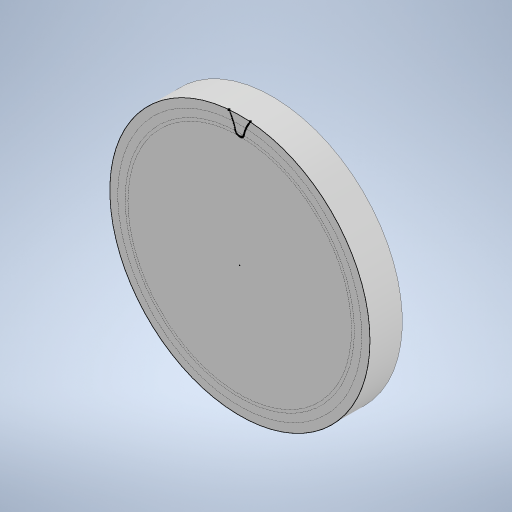
# Autodesk Inventor part: z
Saved by Autodesk Inventor 2024 (Build 280153000, 153)
## iProperties
Created: 2023-10-17
Part Number: z
Material: Generic
Document SubType Name: Modeling
Designer: Kippi
Density: 1 g/cm^3
Appearance: Default
Author: Kippi
Autodesk Inventor part; units mm, degrees
ref_plane "YZ Plane" through (0, 0, 0) normal (1, 0, 0) x (0, 1, 0)
ref_plane "XZ Plane" through (0, 0, 0) normal (0, 1, 0) x (-1, 0, 0)
ref_plane "XY Plane" through (0, 0, 0) normal (0, 0, 1) x (1, 0, 0)
sketch "Sketch1" plane through (0, 0, 0) normal (0, 0, 1) x (1, 0, 0)
  spline S0 degree 3 poles (-6.5259, 79.7334) (-6.2263, 79.2581) (-5.7769, 78.5452) (-5.2243, 77.5668) (-4.8273, 76.8235) (-4.451, 76.0694) (-4.0967, 75.3048) (-3.7666, 74.5294) (-3.4631, 73.7432) (-3.1905, 72.9457) (-2.9506, 72.1376) (-2.7945, 71.4528) (-2.6817, 70.9025) (-2.5626, 70.4977) (-2.4016, 70.1077) (-2.1917, 69.7409) (-1.9706, 69.4668) (-1.7708, 69.2687) (-1.6019, 69.1425) (-1.4288, 69.0215) (-1.2381, 68.9312) (-1.0444, 68.8474) (-0.8391, 68.7979) (-0.6323, 68.7561) (-0.3509, 68.7461) (0, 68.7526) (0.3509, 68.7461) (0.6323, 68.7561) (0.8391, 68.7979) (1.0444, 68.8474) (1.2381, 68.9312) (1.4288, 69.0215) (1.6019, 69.1425) (1.7708, 69.2687) (1.9706, 69.4668) (2.1917, 69.7409) (2.4016, 70.1077) (2.5626, 70.4977) (2.6817, 70.9025) (2.7945, 71.4528) (2.9506, 72.1376) (3.1905, 72.9457) (3.4631, 73.7432) (3.7666, 74.5294) (4.0967, 75.3048) (4.451, 76.0694) (4.8273, 76.8235) (5.2243, 77.5668) (5.7769, 78.5452) (6.2263, 79.2581) (6.5259, 79.7334) knots 0 0 0 0 0.168512 0.252773 0.337035 0.421295 0.505556 0.589816 0.674075 0.758333 0.842588 0.926838 0.968959 1.011074 1.053192 1.095291 1.137378 1.158442 1.179505 1.200561 1.221628 1.242684 1.263747 1.284807 1.305869 1.348 1.390132 1.411193 1.432253 1.453316 1.474372 1.495439 1.516495 1.537558 1.558622 1.60071 1.642808 1.684926 1.727041 1.769162 1.853412 1.937667 2.021925 2.106184 2.190444 2.274705 2.358966 2.443227 2.527488 2.696 2.696 2.696 2.696
  circle A0 centre (0, 0) radius 68.75 construction
  circle A1 centre (0, 0) radius 70.4769 construction
  circle A2 centre (0, 0) radius 75 construction
  circle A3 centre (0, 0) radius 80
  point P0 (-5.6426, 78.2983)
  point P1 (-5.2272, 77.5652)
  point P2 (-4.8307, 76.8217)
  point P3 (-4.4547, 76.0677)
  point P4 (-4.1007, 75.303)
  point P5 (-3.771, 74.5276)
  point P6 (-3.4682, 73.7413)
  point P7 (-3.1959, 72.9439)
  point P8 (-2.9594, 72.1353)
  point P9 (-2.7673, 71.315)
  point P10 (-2.676, 70.9038)
  point P11 (-2.5556, 70.5002)
  point P12 (-2.3934, 70.1115)
  point P13 (-2.1825, 69.7472)
  point P14 (-1.9188, 69.4191)
  point P15 (-1.7676, 69.2724)
  point P16 (-1.6012, 69.1434)
  point P17 (-1.4259, 69.0267)
  point P18 (-1.2376, 68.9322)
  point P19 (-1.0425, 68.8531)
  point P20 (-0.8389, 68.7992)
  point P21 (-0.6316, 68.7618)
  point P22 (-0.4213, 68.7499)
  point P23 (0, 68.75)
  point P24 (0.4213, 68.7499)
  point P25 (0.6316, 68.7618)
  point P26 (0.8389, 68.7992)
  point P27 (1.0425, 68.8531)
  point P28 (1.2376, 68.9322)
  point P29 (1.4259, 69.0267)
  point P30 (1.6012, 69.1434)
  point P31 (1.7676, 69.2724)
  point P32 (1.9188, 69.4191)
  point P33 (2.1825, 69.7472)
  point P34 (2.3934, 70.1115)
  point P35 (2.5556, 70.5002)
  point P36 (2.676, 70.9038)
  point P37 (2.7673, 71.315)
  point P38 (2.9594, 72.1353)
  point P39 (3.1959, 72.9439)
  point P40 (3.4682, 73.7413)
  point P41 (3.771, 74.5276)
  point P42 (4.1007, 75.303)
  point P43 (4.4547, 76.0677)
  point P44 (4.8307, 76.8217)
  point P45 (5.2272, 77.5652)
  point P46 (5.6426, 78.2983)
  constraints: 4 centre point, 2 point on circle, 103 other
extrude "Extrusion1" add sketch "Sketch1" against normal blind 20
equation "\"d0\" = FaceWidth"
equation "\"Module\" = 5"
equation "\"PressureAngle\" = 20deg"
equation "\"UnitProfileClearance\" = 0.25"
equation "\"UnitRoundRadius\" = 0.35"
equation "\"RootDiameter\" = 137.5"
equation "\"BaseDiameter\" = 140.95389"
equation "\"FaceWidth\" = 20"
equation "\"HelixAngle\" = 0"
equation "\"UnitCorrection\" = 0"
equation "\"UnitAddendumModification\" = 0"
equation "\"CircularPitch\" = 15.707963"
equation "\"UnitBacklashShift\" = 0"
equation "\"TotalToolShift\" = 0"
equation "\"IsInternal\" = 0"
body "Solid1"
